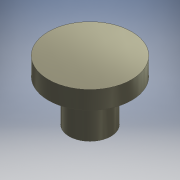
# Autodesk Inventor part: m3 低頭ねじ 3mm (売ってない)
Saved by Autodesk Inventor 2016 (Build 200138000, 138)
## iProperties
Created: 2019-03-17
Part Number: m3 低頭ねじ 3mm (売ってない)
Material: 鋼、炭素鋼
Document SubType Name: Modeling
Designer: mozar
Density: 7.85 g/cm^3
Appearance: ガンメタル
Author: mozar
Autodesk Inventor part; units mm, degrees
ref_plane "YZ Plane" through (0, 0, 0) normal (1, 0, 0) x (0, 1, 0)
ref_plane "XZ Plane" through (0, 0, 0) normal (0, 1, 0) x (-1, 0, 0)
ref_plane "XY Plane" through (0, 0, 0) normal (0, 0, 1) x (1, 0, 0)
sketch "スケッチ1" plane through (0, 0, 0) normal (0, 0, 1) x (1, 0, 0)
  circle A0 centre (0, 0) radius 3
  circle A1 centre (0, 0) radius 1.5
  dimension "d0" = 6
  dimension "d1" = 3
  constraints: 2 centre point, 2 coincident
  measures "d0" diameter of A0
  measures "d1" diameter of A1
extrude "押し出し1" add sketch "スケッチ1" along normal blind 1.3 contours A0 | A1
extrude "押し出し2" add sketch "スケッチ1" against normal blind 3 contours A1
